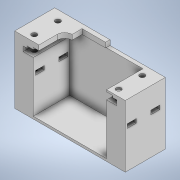
# Autodesk Inventor part: мотор_плеча_2.1
Saved by Autodesk Inventor 2022 (Build 260153000, 153)
## iProperties
Created: 2022-12-03
Part Number: мотор_плеча_2.1
Material: Типовые
Document SubType Name: Modeling
Designer: Папа
Density: 1 g/cm^3
Appearance: По умолчанию
Author: Папа
Autodesk Inventor part; units mm, degrees
sketch "Эскиз1" plane through (0, 0, 0) normal (0, 1, 0) x (-1, 0, 0)
  line L0 (0, 0) -> (-59.05, 0)
  line L1 (-59.05, 0) -> (-59.05, -29.25)
  line L2 (-59.05, -29.25) -> (0, -29.25)
  line L3 (0, -29.25) -> (0, 0)
  line L4 (-74.05, 3) -> (15, 3)
  line L5 (15, 3) -> (15, -32.25)
  line L6 (15, -32.25) -> (-74.05, -32.25)
  line L7 (-74.05, -32.25) -> (-74.05, 3)
  line L8 (-74.05, 3) -> (15, -32.25) construction
  line L9 (15, 3) -> (-74.05, -32.25) construction
  line L10 (0, -29.25) -> (-59.05, 0) construction
  line L11 (0, 0) -> (-59.05, -29.25) construction
  line L12 (15, 0) -> (-74.05, 0)
  point P0 (-29.525, -14.625)
  point P1 (-29.525, -14.625)
  point P2 (-59.05, 0)
  point P3 (-59.05, 0)
  point P4 (0, 0)
  dimension "d0" = 29.25
  dimension "d1" = 59.05
  dimension "d2" = 15
  dimension "d3" = 3
  constraints: 26 end point, 4 midpoint, 4 parallel, 3 point on line, 2 horizontal, 2 perpendicular, 1 collinear
  measures "d0" distance of L2.end L0.start
  measures "d1" distance of L1.end L2.end
  measures "d2" distance between parallel lines of L3 L5
  measures "d3" distance between parallel lines of L6 L2
extrude "Выдавливание1" add sketch "Эскиз1" along normal blind 41 contours L12 L5 L6 L7 L1 L2 L3
sketch "Эскиз2" plane through (0, 0, 0) normal (0, -1, 0) x (1, 0, 0)
  line L0 (74.05, 0) -> (74.05, -32.25) projected
  line L1 (-15, -32.25) -> (-15, 0) projected
  line L2 (74.05, 0) -> (-15, 0)
  line L3 (-15, 0) -> (-15, -32.25)
  line L4 (-15, -32.25) -> (74.05, -32.25)
  line L5 (74.05, -32.25) -> (74.05, 0)
  point P0 (0, 0)
  constraints: 8 end point, 2 parallel, 1 horizontal, 1 perpendicular
extrude "Выдавливание2" add sketch "Эскиз2" along normal blind 2
sketch "Эскиз3" plane through (0, 41, 0) normal (0, 1, 0) x (1, 0, 0)
  circle A0 centre (-4.475, 5.225) radius 2.1
  circle A1 centre (-4.475, 24.225) radius 2.1
  circle A2 centre (63.525, 24.225) radius 2.1
  circle A3 centre (63.525, 5.225) radius 2.1
  line L0 (59.05, 29.25) -> (59.05, 0) construction
  line L1 (0, 0) -> (0, 29.25) construction
  line L2 (59.05, 29.25) -> (0, 29.25) construction
  line L3 (0, 29.25) -> (0, 0.2) construction
  line L4 (0, 0.2) -> (59.05, 0.2) construction
  line L5 (59.05, 0.2) -> (59.05, 29.25) construction
  line L6 (0, 0) -> (59.05, 0) construction
  line L7 (59.05, 0) -> (59.05, 0.2) construction
  line L8 (59.05, 0.2) -> (0, 0.2) construction
  line L9 (0, 0.2) -> (0, 0) construction
  line L10 (0, 0.2) -> (59.05, 29.25) construction
  line L11 (59.05, 0.2) -> (0, 29.25) construction
  line L12 (-4.475, 5.225) -> (63.525, 5.225) construction
  line L13 (63.525, 5.225) -> (63.525, 24.225) construction
  line L14 (63.525, 24.225) -> (-4.475, 24.225) construction
  line L15 (-4.475, 24.225) -> (-4.475, 5.225) construction
  line L16 (-4.475, 5.225) -> (63.525, 24.225) construction
  line L17 (-4.475, 24.225) -> (63.525, 5.225) construction
  point P0 (29.525, 14.725)
  dimension "d8" = 4.2
  dimension "d70" = 0.2
  dimension "d72" = 19
  dimension "d73" = 68
  constraints: 32 end point, 6 parallel, 4 centre point, 3 equal radius, 3 horizontal, 3 perpendicular, 2 coincident, 2 midpoint, 1 point on line
  measures "d8" diameter of A0
  measures "d70" distance between parallel lines of L4 L6
  measures "d72" distance of L13.end A3.centre
  measures "d73" distance of L13.end L14.end
extrude "Выдавливание3" cut sketch "Эскиз3" against normal blind 20
ref_plane "РабПлоскость1" through (0, 31, 0) normal (0, 1, 0) x (1, 0, 0)
sketch "Эскиз4" plane through (0, 31, 0) normal (0, 1, 0) x (1, 0, 0)
  circle A0 centre (63.525, 24.225) radius 2.1 projected
  line L0 (65.589, 27.8) -> (67.6531, 24.225)
  line L1 (67.6531, 24.225) -> (65.589, 20.65)
  line L2 (65.589, 20.65) -> (61.461, 20.65)
  line L3 (61.461, 20.65) -> (59.3969, 24.225)
  line L4 (59.3969, 24.225) -> (61.461, 27.8)
  line L5 (61.461, 27.8) -> (65.589, 27.8)
  circle A1 centre (-4.475, 24.225) radius 2.1 construction
  circle A2 centre (63.525, 5.225) radius 2.1 projected
  line L6 (-4.475, 24.225) -> (63.525, 24.225) construction
  line L7 (63.525, 24.225) -> (63.525, 5.225) construction
  line L8 (63.525, 5.225) -> (-4.475, 5.225) construction
  line L9 (-4.475, 5.225) -> (-4.475, 24.225) construction
  line L10 (-2.411, 27.8) -> (-0.3469, 24.225)
  line L11 (-0.3469, 24.225) -> (-2.411, 20.65)
  line L12 (-2.411, 20.65) -> (-6.539, 20.65)
  line L13 (-6.539, 20.65) -> (-8.6031, 24.225)
  line L14 (-8.6031, 24.225) -> (-6.539, 27.8)
  line L15 (-6.539, 27.8) -> (-2.411, 27.8)
  line L16 (65.589, 8.8) -> (67.6531, 5.225)
  line L17 (67.6531, 5.225) -> (65.589, 1.65)
  line L18 (65.589, 1.65) -> (61.461, 1.65)
  line L19 (61.461, 1.65) -> (59.3969, 5.225)
  line L20 (59.3969, 5.225) -> (61.461, 8.8)
  line L21 (61.461, 8.8) -> (65.589, 8.8)
  line L22 (-2.411, 8.8) -> (-0.3469, 5.225)
  line L23 (-0.3469, 5.225) -> (-2.411, 1.65)
  line L24 (-2.411, 1.65) -> (-6.539, 1.65)
  line L25 (-6.539, 1.65) -> (-8.6031, 5.225)
  line L26 (-8.6031, 5.225) -> (-6.539, 8.8)
  line L27 (-6.539, 8.8) -> (-2.411, 8.8)
  line L28 (65.589, 27.8) -> (74.05, 27.8)
  line L29 (74.05, 32.25) -> (74.05, 0) projected
  line L30 (65.589, 20.65) -> (74.05, 20.65)
  line L31 (29.525, 5.225) -> (29.525, 29.25) construction
  line L32 (0, 29.25) -> (59.05, 29.25) construction
  line L33 (0, 0) -> (0, 29.25) projected
  line L34 (0, 14.625) -> (59.05, 14.625) construction
  line L35 (59.05, 29.25) -> (59.05, 0) projected
  line L36 (59.05, 14.625) -> (0, 14.625) construction
  line L37 (-15, 27.8) -> (-15, 20.65)
  line L38 (-15, 0) -> (-15, 32.25) projected
  line L39 (65.589, 8.8) -> (74.05, 8.8)
  line L40 (65.589, 1.65) -> (74.05, 1.65)
  line L41 (74.05, 1.65) -> (74.05, 8.8)
  line L42 (-2.411, 27.8) -> (0, 27.8)
  line L43 (-2.411, 20.65) -> (0, 20.65)
  line L44 (0, 20.65) -> (0, 27.8)
  line L45 (-2.411, 8.8) -> (0, 8.8)
  line L46 (-2.411, 1.65) -> (0, 1.65)
  line L47 (0, 8.8) -> (0, 1.65)
  point P0 (-4.475, 24.225)
  point P1 (-4.475, 24.225)
  point P2 (63.525, 5.225)
  point P3 (63.525, 5.225)
  point P4 (-4.475, 5.225)
  point P5 (-4.475, 5.225)
  point P6 (-15, 1.45)
  point P7 (-15, 8.6)
  dimension "d14" = 7.15
  dimension "d17" = 68
  dimension "d20" = 19
  constraints: 86 end point, 8 point on line, 7 perpendicular, 6 symmetric about line, 4 collinear, 4 horizontal, 4 midpoint, 3 parallel, 1 coincident, 1 vertical, 55 other
  measures "d14" distance between parallel lines of L1 L4
  measures "d17" distance of point (63.525, 24.225) point (-4.475, 24.225)
  measures "d20" distance of point (63.525, 24.225) point (63.525, 5.225)
extrude "Выдавливание4" cut sketch "Эскиз4" against normal blind 3.25 contours A0 | L28 L29 L30 L1 L0 | L0 L1 L2 L3 L4 L5 | A2 | L42 L33 L43 L11 L10 | L10 L11 L12 L13 L14 L15 | L39 L29 L40 L17 L16 | L16 L17 L18 L19 L20 L21 | L45 L33 L46 L23 L22 | L22 L23 L24 L25 L26 L27
ref_plane "РабПлоскость2" through (0, 19.5, 0) normal (0, -1, 0) x (1, 0, 0)
ref_plane "РабПлоскость3" through (29.525, 41, -32.25) normal (-1, 0, 0) x (0, 0, 1)
ref_plane "РабПлоскость5" through (74.05, 41, 0) normal (0, -1, 0) x (-1, 0, 0)
sketch "Эскиз10" plane through (0, 41, 0) normal (0, 1, 0) x (1, 0, 0)
  line L0 (59.05, 0) -> (74.05, 0) projected
  line L1 (74.05, 32.25) -> (-15, 32.25) projected
  line L2 (74.05, 0) -> (-15, 0)
  line L3 (-15, 0) -> (-15, 32.25)
  line L4 (-15, 32.25) -> (74.05, 32.25)
  line L5 (74.05, 32.25) -> (74.05, 0)
  line L6 (0, 0) -> (0, 29.25) projected
  line L7 (59.05, 29.25) -> (59.05, 0) projected
  line L8 (0, 29.25) -> (59.05, 29.25)
  line L9 (59.05, 29.25) -> (59.05, 0)
  line L10 (59.05, 0) -> (0, 0)
  line L11 (0, 0) -> (0, 29.25)
  circle A0 centre (63.525, 24.225) radius 2.1 projected
  circle A1 centre (63.525, 24.225) radius 2.05
  circle A2 centre (63.525, 5.225) radius 2.05
  circle A3 centre (-4.475, 5.225) radius 2.1 projected
  circle A4 centre (-4.475, 5.225) radius 2.05
  circle A5 centre (-4.475, 24.225) radius 2.05
  circle A6 centre (-4.475, 24.225) radius 2.1 projected
  circle A7 centre (63.525, 5.225) radius 2.1 projected
  point P0 (74.05, 32.25)
  constraints: 16 end point, 6 coincident, 4 centre point, 4 parallel, 2 horizontal, 2 perpendicular
extrude "Выдавливание10" add sketch "Эскиз10" along normal blind 7 contours L7 L8 L6 L2 L3 L1 L5 L0 | A6 | A7
sketch "Эскиз11" plane through (74.05, 41, 0) normal (0, -1, 0) x (-1, 0, 0)
  line L0 (15, 29.25) -> (15, 0) projected
  line L1 (15, 0) -> (6.9, 0)
  line L2 (6.9, 0) -> (6.9, 29.05)
  line L3 (6.9, 29.05) -> (15, 29.05)
  line L4 (15, 29.05) -> (15, 0)
  point P0 (74.05, 0)
  point P1 (15, 29.05)
  dimension "d61" = 8.1
  constraints: 8 end point, 2 parallel, 1 horizontal, 1 perpendicular
  measures "d61" distance between parallel lines of L0 L2
extrude "Выдавливание11" cut sketch "Эскиз11" against normal blind 4
fillet "Сопряжение8" radius 1.95 1 edges at (67.15, 43, -29.05)
sketch "Эскиз13" plane through (74.05, 45, 0) normal (0, -1, 0) x (1, 0, 0)
  line L0 (-15, -29.25) -> (-15, 0) projected
  line L1 (-74.05, -29.25) -> (-15, -29.25) projected
  line L2 (-15, 0) -> (-15, -29.25)
  line L3 (-20, -13.625) -> (-10, -13.625)
  line L4 (-10, -13.625) -> (-10, -15.625)
  line L5 (-10, -15.625) -> (-20, -15.625)
  line L6 (-20, -15.625) -> (-20, -13.625)
  line L7 (-20, -13.625) -> (-10, -15.625) construction
  line L8 (-10, -13.625) -> (-20, -15.625) construction
  arc A0 (-11, -15.625) -> (-11, -13.625) centre (-11, -14.625) ccw
  line L9 (-10, -14.625) -> (-15, -14.625)
  line L10 (-15, -14.625) -> (-15, 0)
  line L11 (-15, 0) -> (-10, 0)
  line L12 (-10, 0) -> (-10, -14.625)
  point P0 (-74.05, 0)
  point P1 (-15, -13.625)
  dimension "d65" = 10
  dimension "d66" = 2
  constraints: 22 end point, 4 parallel, 3 midpoint, 3 point on circle, 3 tangent, 2 horizontal, 2 perpendicular, 2 point on line, 1 centre point, 1 vertical
  measures "d65" distance of L4.end L5.end
  measures "d66" distance of L3.end L4.end
extrude "Выдавливание12" cut sketch "Эскиз13" against normal blind 1.5
fillet "Сопряжение9" radius 1 1 edges at (64.05, 45.75, -15.625)
mirror "Зеркальное отражение2" about plane through (29.525, 41, -32.25) normal (-1, 0, 0) of "Выдавливание11", "Выдавливание12", "Сопряжение9"
sketch "Эскиз15" plane through (0, 48, 0) normal (0, 1, 0) x (1, 0, 0)
  arc A0 (42.1128, 0.625) -> (42.1128, 28.725) centre (44.775, 14.675) ccw
  line L0 (42.1128, 28.725) -> (10.5328, 28.725)
  line L1 (10.5328, 0.625) -> (42.1128, 0.625)
  arc A1 (10.5328, 20.7) -> (10.5328, 8.65) centre (10.5328, 14.675) ccw
  line L2 (10.5328, 28.725) -> (10.5328, 20.7)
  line L3 (10.5328, 8.65) -> (10.5328, 0.625)
  line L4 (-7.975, 29.225) -> (67.025, 29.225)
  line L5 (67.025, 29.225) -> (67.025, 0.125)
  line L6 (67.025, 0.125) -> (-7.975, 0.125)
  line L7 (-7.975, 0.125) -> (-7.975, 29.225)
  line L8 (-7.975, 29.225) -> (67.025, 0.125) construction
  line L9 (67.025, 29.225) -> (-7.975, 0.125) construction
  line L10 (59.075, 14.675) -> (67.025, 14.675)
  line L11 (10.5328, 20.7) -> (10.5328, 8.65) construction
  line L12 (67.025, 0.125) -> (-7.975, 0.125)
  line L13 (-7.975, 0.125) -> (-7.975, -2.875)
  line L14 (-7.975, -2.875) -> (67.025, -2.875)
  line L15 (67.025, -2.875) -> (67.025, 0.125)
  circle A2 centre (63.525, 24.225) radius 2.05
  circle A3 centre (63.525, 24.225) radius 2.1 projected
  circle A4 centre (-4.475, 24.225) radius 2.1 projected
  circle A5 centre (-4.475, 24.225) radius 2.1
  circle A6 centre (-4.475, 5.225) radius 2.1 projected
  circle A7 centre (-4.475, 5.225) radius 2.1
  circle A8 centre (63.525, 5.225) radius 2.05 projected
  circle A9 centre (63.525, 5.225) radius 2.05
  line L16 (4.5078, 14.675) -> (4.5078, 0)
  line L17 (59.05, 0) -> (0, 0) projected
  line L18 (29.525, 14.675) -> (29.525, 0)
  line L19 (74.05, 32.25) -> (-15, 32.25) projected
  line L20 (-15, 32.25) -> (29.525, 32.25)
  line L21 (29.525, 32.25) -> (29.525, 0)
  line L22 (29.525, 0) -> (-15, 0)
  line L23 (-15, 0) -> (-15, 32.25)
  point P0 (-52.75, -14.55)
  point P1 (29.525, 32.25)
  point P2 (-7.975, 0)
  point P3 (-7.975, 0.125)
  point P4 (4.5078, 0.125)
  point P5 (29.525, 28.725)
  dimension "d75" = 28.6
  dimension "d76" = 12.05
  dimension "d77" = 31.58
  dimension "d79" = 29.1
  dimension "d80" = 75
  dimension "d81" = 3
  dimension "d82" = 22.25
  dimension "d83" = 3.5
  dimension "d84" = 5
  dimension "d85" = 4.1
  dimension "d86" = 7.95
  dimension "d87" = 28.1
  constraints: 44 end point, 8 parallel, 6 centre point, 6 coincident, 6 point on circle, 5 horizontal, 5 perpendicular, 4 collinear, 4 midpoint, 1 point on line, 1 vertical
  measures "d75" diameter of A0
  measures "d76" diameter of A1
  measures "d77" distance of L1.start L1.end
  measures "d79" distance between parallel lines of L4 L6
  measures "d80" distance of L5.end L6.end
  measures "d81" distance of L14.end L5.end
  measures "d82" distance from line of L5 point (44.775, 14.675)
  measures "d83" distance from line of L5 A2.centre
  measures "d84" distance from line of L4 A2.centre
  measures "d85" diameter of A2
  measures "d86" distance of L10.start L10.end
  measures "d87" distance between parallel lines of L1 L0
extrude "Выдавливание13" add sketch "Эскиз15" along normal blind 4 contours L0 L2 A1 L16 L6 L7 L4 L21 | L16 L17 L22 L13 L6 | L4 L7 L13 L22 L23 L19 L21
